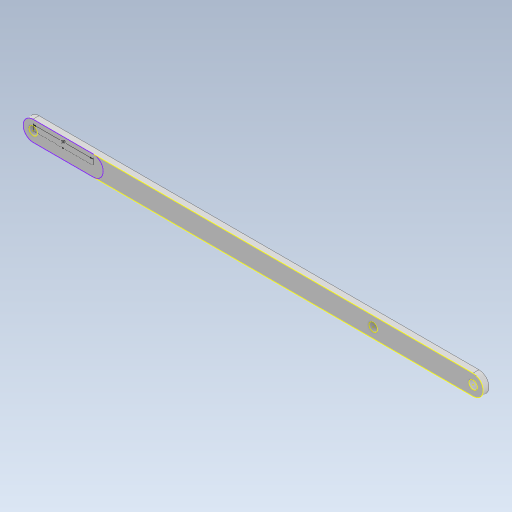
# Autodesk Inventor part: adjustable_130
Saved by Autodesk Inventor 2023 (Build 270158000, 158)
## iProperties
Created: 2023-04-16
Part Number: adjustable_130
Material: 一般
Document SubType Name: Modeling
Designer: JOU
Density: 1 g/cm^3
Appearance: 預設
Author: JOU
Autodesk Inventor part; units mm, degrees
ref_plane "YZ Plane" through (0, 0, 0) normal (1, 0, 0) x (0, 1, 0)
ref_plane "XZ Plane" through (0, 0, 0) normal (0, 1, 0) x (-1, 0, 0)
ref_plane "XY Plane" through (0, 0, 0) normal (0, 0, 1) x (1, 0, 0)
sketch "草圖1" plane through (0, 0, 0) normal (0, 0, 1) x (1, 0, 0)
  line L0 (-220, 0) -> (0, 0) construction
  line L1 (-220, -5) -> (0, -5)
  line L2 (0, 5) -> (-220, 5)
  arc A0 (-220, 5) -> (-220, -5) centre (-220, 0) ccw
  arc A1 (0, -5) -> (0, 5) centre (0, 0) ccw
  circle A2 centre (-220, 0) radius 2.1
  circle A3 centre (0, 0) radius 2.1
  circle A4 centre (-50, 0) radius 2.1
  point P0 (-110, 0)
  dimension "d0" = 220
  dimension "d1" = 10
  dimension "d2" = 4.2
  dimension "d3" = 4.2
  dimension "d23" = 170
  constraints: 8 end point, 5 centre point, 4 point on circle, 4 tangent, 3 coincident, 1 equal radius, 1 horizontal, 1 midpoint, 1 parallel, 1 point on line
  measures "d0" distance of L2.start L2.end
  measures "d1" distance between parallel lines of L1 L2
  measures "d2" diameter of A2
  measures "d3" diameter of A3
  measures "d23" distance of A2.centre A4.centre
extrude "擠出1" add sketch "草圖1" along normal blind 3
sketch "草圖5" plane through (0, 0, 3) normal (0, 0, 1) x (1, 0, 0)
  arc A0 (0, -5) -> (0, 5) centre (0, 0) ccw projected
  line L0 (0, 5) -> (-220, 5) projected
  arc A1 (-220, 5) -> (-220, -5) centre (-220, 0) ccw projected
  line L1 (-220, -5) -> (0, -5) projected
  circle A2 centre (-50, 0) radius 2.1 projected
  circle A3 centre (0, 0) radius 2.1 projected
  circle A4 centre (-220, 0) radius 2.1 projected
  circle A5 centre (-220, 0) radius 2.1 projected
  line L2 (-220, 0) -> (-190, 0) construction
  line L3 (-220, -5) -> (-190, -5)
  line L4 (-190, 5) -> (-220, 5)
  arc A6 (-220, 5) -> (-220, -5) centre (-220, 0) ccw
  arc A7 (-190, -5) -> (-190, 5) centre (-190, 0) ccw
  point P0 (-205, 0)
  dimension "d24" = 30
  constraints: 8 end point, 4 point on circle, 4 tangent, 2 centre point, 1 horizontal, 1 midpoint, 1 parallel
  measures "d24" distance of L2.start L2.end
